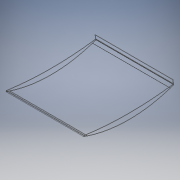
# Autodesk Inventor part: element_gurnee
Saved by Autodesk Inventor 2018.1 (Build 221171000, 171)
## iProperties
Created: 2017-10-18
Part Number: element_gurnee
Material: CFRP
Document SubType Name: Modeling
Designer: kuwano
Density: 1.43 g/cm^3
Appearance: カーボンファイバー
Mass: 137.207 g
Surface Area: 1928.57 cm^2
Volume: 95.949 cm^3
Author: kuwano
Autodesk Inventor part; units mm, degrees
ref_plane "YZ Plane" through (0, 0, 0) normal (1, 0, 0) x (0, 1, 0)
ref_plane "XZ Plane" through (0, 0, 0) normal (0, 1, 0) x (-1, 0, 0)
ref_plane "XY Plane" through (0, 0, 0) normal (0, 0, 1) x (1, 0, 0)
sketch "スケッチ1" plane through (0, 0, 0) normal (1, 0, 0) x (0, 1, 0)
  arc A0 (20.4585, 116.0261) -> (20.4585, -116.0261) centre (339.2375, 0) ccw
  line L0 (23.2776, 115) -> (20.4585, 116.0261)
  line L1 (23.2776, -115) -> (20.4585, -116.0261)
  line L2 (0, -162.4365) -> (0, 162.4365) projected
  arc A1 (23.2776, 115) -> (23.2776, -115) centre (836.8483, 0) ccw
  point P0 (0, 0)
  point P1 (0, 0)
  dimension "d0" = 3
  dimension "d1" = 230
  dimension "d2" = 40
  dimension "d12" = 3
  constraints: 5 point on circle, 4 end point, 2 centre point, 2 line through centre, 1 coincident, 1 tangent
  measures "d0" distance of L0.start L0.end
  measures "d1" distance of L1.start L0.start
  measures "d2" angle of L1 L0
  measures "d12" distance of L1.start L1.end
extrude "押し出し1" add sketch "スケッチ1" along normal blind 200
sketch "スケッチ2" plane through (0, 0, 0) normal (-1, 0, 0) x (0, 0, 1)
  line L0 (-116.0261, 20.4585) -> (-106.5797, 17.1772)
  arc A0 (-116.0261, 20.4585) -> (116.0261, 20.4585) centre (0, 339.2375) ccw projected
  line L1 (0, 0) -> (0, -168.7214)
  line L2 (116.0261, 20.4585) -> (106.5797, 17.1772)
  arc A1 (-116.0261, 20.4585) -> (116.0261, 20.4585) centre (0, 339.2375) ccw
  point P0 (-116.0261, 20.4585)
  dimension "d13" = 10
  constraints: 6 end point, 4 point on circle, 4 symmetric about line, 2 coincident, 1 centre point, 1 vertical, 1 other
  measures "d13" distance of L0.start L0.end
extrude "押し出し2" cut sketch "スケッチ2" against normal through all
shell "シェル1" thickness 1 removed faces 2 at (0, 10.498, -16.8297) at (200, 10.498, -16.8297)
sketch "スケッチ6" plane through (200, 0, 0) normal (1, 0, 0) x (0, 0, -1)
  arc A0 (-115, 23.2776) -> (115, 23.2776) centre (0, 836.8483) ccw projected
  line L0 (115, 23.2776) -> (113.6004, 33.1792)
  line L1 (113.6004, 33.1792) -> (112.6102, 33.0392)
  line L2 (112.6102, 33.0392) -> (114.0098, 23.1382)
  point P0 (0, 0)
  dimension "d18" = 1
  dimension "d19" = 10
  constraints: 6 end point, 2 perpendicular, 1 line through centre, 1 point on circle
  measures "d18" distance of L0.end L1.end
  measures "d19" distance of L0.start L0.end
extrude "押し出し5" add sketch "スケッチ6" against normal blind 200
